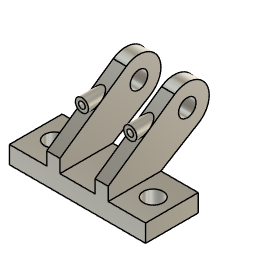
exercises01 (Autodesk Fusion 360 design; units mm, degrees)
Autodesk Fusion 360 part; units mm, degrees
sketch "草图1" plane through (0, 0, 0) normal (0, 0, 1) x (1, 0, 0)
  line L0 (-31, 12) -> (31, 12)
  line L1 (31, 12) -> (31, -12)
  line L2 (31, -12) -> (-31, -12)
  line L3 (-31, -12) -> (-31, 12)
  circle A0 centre (-22.5, 0) radius 4.5
  circle A1 centre (22.5, 0) radius 4.5
  line L4 (0, 20) -> (0, -25) construction
  line L5 (35, 0) -> (-34, 0) construction
  dimension "d1" = 24
  dimension "d2" = 62
  dimension "d3" = 9
  dimension "d4" = 45
  constraint horizontal L0
  constraint vertical L1
  constraint horizontal L2
  constraint vertical L3
  constraint perpendicular L2 L4
  constraint horizontal L5
  constraint symmetric L1 L3 L4
  constraint symmetric L0 L2 L5
  constraint symmetric A0.centre A1.centre L4
  constraint equal A0 A1
  constraint coincident A0.centre L5
  measures "d1" distance of L0.end L1.end
  measures "d2" distance of L1.end L2.end
  measures "d3" diameter of A0
  measures "d4" distance of A0.centre A1.centre
extrude "拉伸1" add sketch "草图1" against normal blind 8 makes body 1
ref_plane "工作平面1" through (-14, 0, -4) normal (-1, 0, 0) x (0, 1, 0)
sketch "草图2" plane through (-14, 0, 0) normal (-1, 0, 0) x (0, -1, 0)
  line L0 (-12, 0) -> (12, 0)
  line L1 (12, 0) -> (12, 6)
  line L2 (12, 6) -> (-18.2642, 27.1915)
  line L3 (-12, 0) -> (-29.1954, 10.4555)
  arc A0 (-18.2642, 27.1915) -> (-29.1954, 10.4555) centre (-24, 19) ccw
  circle A1 centre (-24, 19) radius 4
  line L4 (0, 23) -> (0, -19) construction
  line L5 (12, -8) -> (-12, -8) construction
  line L6 (12, 0) -> (12, -8) construction
  dimension "d8" = 6
  dimension "d9" = 27
  dimension "d10" = 36
  dimension "d11" = 8
  dimension "d12" = 10
  dimension "d13" = 24
  constraint horizontal L0
  constraint perpendicular L0 L1
  constraint vertical L4
  constraint coincident A0.centre A1.centre
  constraint tangent L2 A0
  constraint tangent L3 A0
  constraint symmetric L0.start L4 L0.end
  measures "d8" distance of L0.end L1.end
  measures "d9" distance of A0.centre L5
  measures "d10" distance of A0.centre L6
  measures "d11" diameter of A1
  measures "d12" radius of A0
  measures "d13" distance of L0.start L0.end
extrude "拉伸2" add sketch "草图2" against normal blind 6 separate body makes body 2
ref_plane "工作平面2" through (-11, 1, 3) normal (0, -1, 0) x (0, 0, -1)
sketch "草图3" plane through (0, 1, 0) normal (0, -1, 0) x (-1, 0, 0)
  circle A0 centre (11, -19) radius 3
  circle A1 centre (11, -19) radius 1.5
  line L0 (-31, 8) -> (31, 8)
  line L1 (8, -27.1915) -> (8, -6)
  dimension "d17" = 6
  dimension "d18" = 3
  dimension "d19" = 27
  dimension "d20" = 3
  constraint concentric A0 A1
  measures "d17" diameter of A0
  measures "d18" diameter of A1
  measures "d19" distance of A0.centre L0
  measures "d20" distance of A0.centre L1
extrude "拉伸3" add sketch "草图3" along normal up to surface end surface at (-10, 20.005, 18.8006) on bodies 2 bodies 2
extrude "拉伸4" cut sketch "草图3" along normal up to surface contours A1 end surface at (-10, 20.005, 18.8006) on bodies 2 bodies 2
copy_body "复制和粘贴实体1" bodies 2 makes body 3
move_body "移动1" bodies 3 to x (1, 0, 0) y (0, 1, 0) z (0, 0, 1) at (22, 0, 0)
combine "合并1" operation add target body 1 tool bodies 3 2
